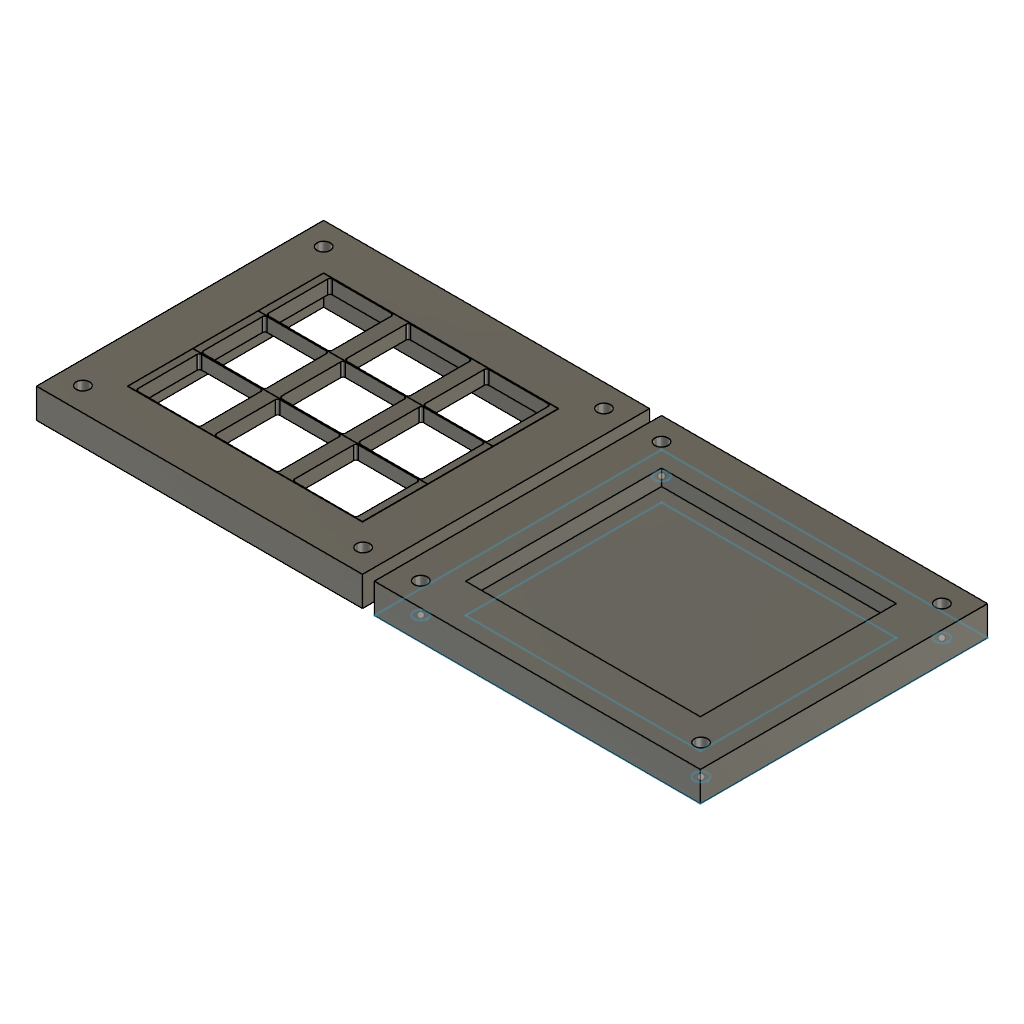
NumPad (Autodesk Fusion 360 design; units mm, degrees)
part number: 2026-09-25-08-35-41-918
Autodesk Fusion 360 part; units mm, degrees
sketch "Sketch1" plane through (0, 0, 0) normal (0, 0, 1) x (1, 0, 0)
  line L0 (-25, 25) -> (26.4, 25)
  line L1 (26.4, 25) -> (26.4, -17.9)
  line L2 (26.4, -17.9) -> (-25, -17.9)
  line L3 (-25, -17.9) -> (-25, 25)
  line L4 (-35, 35) -> (36.4, 35)
  line L5 (36.4, 35) -> (36.4, -27.9)
  line L6 (36.4, -27.9) -> (-35, -27.9)
  line L7 (-35, -27.9) -> (-35, 35)
  circle A0 centre (-30, 30) radius 1.45
  circle A1 centre (-30, -22.7212) radius 1.45
  circle A2 centre (31.3768, 30) radius 1.45
  circle A3 centre (31.3768, -22.7212) radius 1.45
  dimension "d1" = 51.4
  dimension "d2" = 42.9
  dimension "d3" = 71.4
  dimension "d4" = 62.9
  dimension "d5" = 2.9
  dimension "d6" = 10
  dimension "d7" = 2.9
  dimension "d8" = 2.9
  dimension "d9" = 2.9
  constraint horizontal L0
  constraint vertical L1
  constraint horizontal L2
  constraint vertical L3
  constraint horizontal L4
  constraint vertical L5
  constraint horizontal L6
  constraint vertical L7
  measures "d1" distance of L0.start L0.end
  measures "d2" distance of L0.start L2.end
  measures "d3" distance of L4.start L4.end
  measures "d4" distance of L4.start L6.end
  measures "d5" diameter of A0
  measures "d6" distance of L0.end L5
  measures "d7" diameter of A1
  measures "d8" diameter of A2
  measures "d9" diameter of A3
extrude "Extrude1" add sketch "Sketch1" along normal blind 3 contours L0 L1 L2 L3 | L4 L5 L6 L7 makes body 1
extrude "Extrude2" cut sketch "Sketch1" along normal blind 11 contours L0 L1 L2 L3 | L4 L5 L6 L7 | A0 | A1 | A2 | A3 bodies 1
extrude "Extrude3" add sketch "Sketch1" along normal blind 3 contours L0 L1 L2 L3 bodies 1
extrude "Extrude4" add sketch "Sketch1" along normal blind 13 bodies 1
sketch "plate-2026-09-24T23_36_53.372Z" plane through (0, 0, 3) normal (0, 0, 1) x (1, 0, 0)
  line L0 (-22.9113, -3.7982) -> (-9.9113, -3.7982)
  line L1 (-22.9113, -17.7982) -> (-9.9113, -17.7982)
  line L2 (-23.4113, -4.2982) -> (-23.4113, -17.2982)
  line L3 (-9.4113, -4.2982) -> (-9.4113, -17.2982)
  arc A0 (-22.9113, -3.7982) -> (-23.4113, -4.2982) centre (-22.9113, -4.2982) ccw
  arc A1 (-9.4113, -4.2982) -> (-9.9113, -3.7982) centre (-9.9113, -4.2982) ccw
  arc A2 (-23.4113, -17.2982) -> (-22.9113, -17.7982) centre (-22.9113, -17.2982) ccw
  arc A3 (-9.9113, -17.7982) -> (-9.4113, -17.2982) centre (-9.9113, -17.2982) ccw
  line L4 (-5.7613, -3.7982) -> (7.2387, -3.7982)
  line L5 (-5.7613, -17.7982) -> (7.2387, -17.7982)
  line L6 (-6.2613, -4.2982) -> (-6.2613, -17.2982)
  line L7 (7.7387, -4.2982) -> (7.7387, -17.2982)
  arc A4 (-5.7613, -3.7982) -> (-6.2613, -4.2982) centre (-5.7613, -4.2982) ccw
  arc A5 (7.7387, -4.2982) -> (7.2387, -3.7982) centre (7.2387, -4.2982) ccw
  arc A6 (-6.2613, -17.2982) -> (-5.7613, -17.7982) centre (-5.7613, -17.2982) ccw
  arc A7 (7.2387, -17.7982) -> (7.7387, -17.2982) centre (7.2387, -17.2982) ccw
  line L8 (11.3887, -3.7982) -> (24.3887, -3.7982)
  line L9 (11.3887, -17.7982) -> (24.3887, -17.7982)
  line L10 (10.8887, -4.2982) -> (10.8887, -17.2982)
  line L11 (24.8887, -4.2982) -> (24.8887, -17.2982)
  arc A8 (11.3887, -3.7982) -> (10.8887, -4.2982) centre (11.3887, -4.2982) ccw
  arc A9 (24.8887, -4.2982) -> (24.3887, -3.7982) centre (24.3887, -4.2982) ccw
  arc A10 (10.8887, -17.2982) -> (11.3887, -17.7982) centre (11.3887, -17.2982) ccw
  arc A11 (24.3887, -17.7982) -> (24.8887, -17.2982) centre (24.3887, -17.2982) ccw
  line L12 (-24.9863, -17.9482) -> (26.4637, -17.9482)
  line L13 (-24.9863, -3.6482) -> (26.4637, -3.6482)
  line L14 (-24.9863, -17.9482) -> (-24.9863, -3.6482)
  line L15 (26.4637, -17.9482) -> (26.4637, -3.6482)
extrude "Extrude5" add sketch "plate-2026-09-24T23_36_53.372Z" along normal blind 3 separate body makes body 2
move_body "Move1" bodies 2 to x (1, 0, 0) y (0, 1, 0) z (0, 0, 1) at (0, 0, 7)
copy_body "CopyPasteBodies1" bodies 2 makes body 3
move_body "Move2" bodies 3 to x (1, 0, 0) y (0, 1, 0) z (0, 0, 1) at (0, 14.22, 0)
copy_body "CopyPasteBodies2" bodies 2 makes body 4
move_body "Move3" bodies 4 to x (1, 0, 0) y (0, 1, 0) z (0, 0, 1) at (0, 28.6, 0)
move_body "Move4" bodies 3 to x (1, 0, 0) y (0, 1, 0) z (0, 0, 1) at (0, 0.1, 0)
split "Split1" by plane through (0.7, 3.55, 6.5) normal (0, 0, 1) bodies 1 makes body 5 at (-28.8167, 10.7596, 13)
move_body "Move5" bodies 2 3 4 5 to x (1, 0, 0) y (0, 1, 0) z (0, 0, 1) at (-74, 0, -6)
move_body "Move6" bodies 5 4 3 2 to x (1, 0, 0) y (0, 1, 0) z (0, 0, 1) at (0, 0, -0.5)
